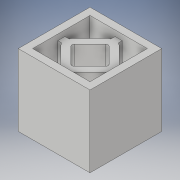
# Autodesk Inventor part: Axle beam base-linear
Saved by Autodesk Inventor 2019.3 (Build 233278000, 278)
## iProperties
Created: 2019-01-29
Part Number: Axle beam base-linear
Material: Generic
Document SubType Name: Modeling
Designer: Varga Daniel
Density: 1 g/cm^3
Appearance: Default
Hole_height: 8,400 mm
Author: Varga Daniel
Autodesk Inventor part; units mm, degrees
ref_plane "YZ Plane" through (0, 0, 0) normal (1, 0, 0) x (0, 1, 0)
ref_plane "XZ Plane" through (0, 0, 0) normal (0, 1, 0) x (-1, 0, 0)
derived "Base_part.ipt"
sketch "Beam_sketch" plane through (0, 0, 0) normal (0, 1, 0) x (-1, 0, 0)
  line L0 (5, 0) -> (25, 0)
  line L1 (30, 5) -> (30, 25)
  line L2 (25, 30) -> (5, 30)
  line L3 (0, 25) -> (0, 5)
  line L4 (5, 29) -> (25, 29)
  line L5 (29, 25) -> (29, 5)
  line L6 (25, 1) -> (5, 1)
  line L7 (1, 5) -> (1, 25)
  circle A0 centre (5, 5) radius 2.5
  circle A1 centre (5, 5) radius 3.5
  arc A2 (25, 0) -> (30, 5) centre (25, 5) ccw
  arc A3 (30, 25) -> (25, 30) centre (25, 25) ccw
  arc A4 (5, 30) -> (0, 25) centre (5, 25) ccw
  arc A5 (0, 5) -> (5, 0) centre (5, 5) ccw
  arc A6 (1, 5) -> (5, 1) centre (5, 5) ccw
  arc A7 (5, 29) -> (1, 25) centre (5, 25) ccw
  arc A8 (29, 25) -> (25, 29) centre (25, 25) ccw
  arc A9 (25, 1) -> (29, 5) centre (25, 5) ccw
  line L8 (49.1041, 15) -> (-27.081, 15) construction
  line L9 (31.1478, 10) -> (-2.4877, 10) construction
  line L10 (-2.8604, 5) -> (35.495, 5) construction
  line L11 (5, -2.5736) -> (5, 36.7522) construction
  line L12 (15, -1.4978) -> (15, 34.8784) construction
  line L13 (1.5359, 5.5) -> (1, 5.5)
  line L14 (1.5359, 4.5) -> (1.0314, 4.5)
  line L15 (28.9686, 4.5) -> (8.4641, 4.5)
  line L16 (29, 5.5) -> (8.4641, 5.5)
  line L17 (4.5, 1.5359) -> (4.5, 1.0314)
  line L18 (5.5, 1.5359) -> (5.5, 1)
  line L19 (29, 10.5) -> (1, 10.5)
  line L20 (29, 9.5) -> (1, 9.5)
  line L21 (4.5, 28.9686) -> (4.5, 10.5)
  line L22 (4.5, 9.5) -> (4.5, 8.4641)
  line L23 (5.5, 29) -> (5.5, 10.5)
  line L24 (5.5, 9.5) -> (5.5, 8.4641)
  point P0 (0, 0)
  point P1 (30, 30)
  point P2 (0, 30)
sketch "Axle_hole_sketch" plane through (0, 0, 0) normal (0, 1, 0) x (-1, 0, 0)
  line L0 (-14.3207, 2.4447) -> (-17.4707, 2.4447)
  line L1 (-17.7707, 2.7447) -> (-17.7707, 5.8947)
  line L2 (-17.4707, 6.1947) -> (-14.3207, 6.1947)
  line L3 (-14.0207, 5.8947) -> (-14.0207, 2.7447)
  line L4 (-14.0207, 2.4447) -> (-17.7707, 6.1947) construction
  line L5 (-17.7707, 2.4447) -> (-14.0207, 6.1947) construction
  arc A0 (-14.3207, 2.4447) -> (-14.0207, 2.7447) centre (-14.3207, 2.7447) ccw
  arc A1 (-17.7707, 2.7447) -> (-17.4707, 2.4447) centre (-17.4707, 2.7447) ccw
  arc A2 (-17.4707, 6.1947) -> (-17.7707, 5.8947) centre (-17.4707, 5.8947) ccw
  arc A3 (-14.0207, 5.8947) -> (-14.3207, 6.1947) centre (-14.3207, 5.8947) ccw
  point P0 (0, 0)
  point P1 (-15.8957, 4.3197)
  dimension "d142" = 3.75
  dimension "d143" = 3.75
  dimension "d144" = 0.3
  measures "d142" distance between parallel lines of L3 L1
  measures "d143" distance between parallel lines of L2 L0
  measures "d144" radius of A3
sketch "Sketch2" plane through (0, 0, 0) normal (0, 1, 0) x (-1, 0, 0)
  circle A0 centre (5, 5) radius 2.5 construction
  circle A1 centre (5, 5) radius 3.5 construction
  line L0 (9.2761, 0) -> (-0.5, 0) construction
  line L1 (0, 4.8106) -> (0, -6.1444) construction
  line L2 (5, 0) -> (-0.5, 0)
  line L3 (5, 0) -> (5, -10)
  line L4 (5, -10) -> (-5, -10)
  line L5 (-5, -10) -> (-5, -4.5)
  line L6 (5, -5) -> (-5, -5) construction
  line L7 (3.4274, -5.5) -> (4, -5.5)
  line L8 (3.4274, -4.5) -> (4, -4.5)
  line L9 (-3.4274, -4.5) -> (-4, -4.5)
  line L10 (-3.4274, -5.5) -> (-4, -5.5)
  line L11 (0.5, -1.5726) -> (0.5, -1)
  line L12 (-0.5, -1.5726) -> (-0.5, -1)
  line L13 (0.5, -9) -> (0.5, -8.4274)
  line L14 (-0.5, -8.4274) -> (-0.5, -9)
  line L15 (2.4395, -5.2121) -> (0.2121, -7.4395)
  line L16 (-0.2121, -7.4395) -> (-2.4395, -5.2121)
  line L17 (-2.4395, -4.7879) -> (-0.2121, -2.5605)
  line L18 (0.2121, -2.5605) -> (2.4395, -4.7879)
  line L19 (2.6517, -5) -> (-2.6517, -5) construction
  line L20 (0, -7.6517) -> (0, -2.3483) construction
  arc A2 (-0.2121, -7.4395) -> (0.2121, -7.4395) centre (0, -7.2274) ccw
  arc A3 (-2.4395, -4.7879) -> (-2.4395, -5.2121) centre (-2.2274, -5) ccw
  arc A4 (0.2121, -2.5605) -> (-0.2121, -2.5605) centre (0, -2.7726) ccw
  arc A5 (2.4395, -5.2121) -> (2.4395, -4.7879) centre (2.2274, -5) ccw
  line L21 (-0.9192, -1.8534) -> (-3.1466, -4.0808)
  arc A6 (-3.1466, -4.0808) -> (-3.1466, -5.9192) centre (-2.2274, -5) ccw
  line L22 (-3.1466, -5.9192) -> (-0.9192, -8.1466)
  arc A7 (-0.9192, -8.1466) -> (0.9192, -8.1466) centre (0, -7.2274) ccw
  line L23 (0.9192, -8.1466) -> (3.1466, -5.9192)
  arc A8 (3.1466, -5.9192) -> (3.1466, -4.0808) centre (2.2274, -5) ccw
  line L24 (3.1466, -4.0808) -> (0.9192, -1.8534)
  arc A9 (0.9192, -1.8534) -> (-0.9192, -1.8534) centre (0, -2.7726) ccw
  line L25 (-0.5, 0) -> (-4, 0)
  line L26 (-4, 0) -> (-5, 0)
  line L27 (-0.5, 0) -> (-6.9818, 0) construction
  line L28 (-5, -1) -> (-5, 0)
  line L29 (-5, -4.5) -> (-5, -1)
  line L30 (5, -9) -> (-5, -9)
  line L31 (-5, -1) -> (5, -1)
  line L32 (4, -9) -> (4, -1)
  line L33 (-4, -1) -> (-4, -9)
  point P0 (0, 0)
  point P1 (4, -10)
  point P2 (-4, -10)
  point P3 (5, -5.5)
  point P4 (5, -4.5)
  point P5 (-5, -5.5)
  point P6 (0.5, 0)
  point P7 (0.5, -10)
  point P8 (-0.5, -10)
  point P9 (4, 0)
  point P10 (0, -5)
  dimension "d105" = 5
  dimension "d106" = 7
  dimension "d127" = 5
  dimension "d128" = 5
  dimension "d130" = 10
  dimension "d134" = 1
  dimension "d135" = 1
  dimension "d147" = 3.75
  dimension "d148" = 0.3
  dimension "d149" = 1
  dimension "d161" = 1
  dimension "d162" = 1
  dimension "d163" = 1
  dimension "d164" = 1
  constraints: 69 end point, 39 point on line, 24 point on circle, 15 perpendicular, 11 collinear, 10 parallel, 8 centre point, 8 tangent, 4 midpoint, 3 equal radius, 2 horizontal, 2 vertical, 10 other
  measures "d105" diameter of A0
  measures "d106" diameter of A1
  measures "d127" distance between parallel lines of L3 L1
  measures "d128" distance between parallel lines of L5 L1
  measures "d130" distance between parallel lines of L4 L2
  measures "d134" distance between parallel lines of L8 L7
  measures "d135" distance between parallel lines of L12 L11
  measures "d147" distance between parallel lines of L15 L17
  measures "d148" radius of A2
  measures "d149" distance between parallel lines of L21 L17
  measures "d161" distance between parallel lines of L4 L30
  measures "d162" distance between parallel lines of L2 L31
  measures "d163" distance between parallel lines of L32 L3
  measures "d164" distance between parallel lines of L29 L33
ref_plane "Work Plane2" through (-5, 0, 0) normal (0, 1, 0) x (1, 0, 0)
extrude "Extrusion19" add sketch "Sketch2" along normal mid plane 8.4 contours L11 A9 L12 L31 | L32 L7 A8 L8 | L30 L14 A7 L13 | A9 L24 A8 L23 A7 L22 A6 L21 | L9 A6 L10 L33
extrude "Extrusion21" add sketch "Sketch2" along normal mid plane 1 contours L32 L8 A8 L24 A9 L11 L31 | L30 L13 A7 L23 A8 L7 L32 | A9 L24 A8 L23 A7 L22 A6 L21 | L12 A9 L21 A6 L9 L33 L31 | L30 L33 L10 A6 L22 A7 L14
extrude "Extrusion24" add sketch "Sketch2" along normal mid plane 10 contours L3 L31 L28 L26 L25 L2 | L3 L30 L32 L31 | L3 L4 L5 L30 | L31 L33 L30 L5 L29
body "Solid5"
